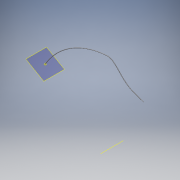
# Autodesk Inventor part: bumper_wire
Saved by Autodesk Inventor 2016 (Build 200138000, 138)
## iProperties
Created: 2016-02-23
Part Number: bumper_wire
Material: Generic
Document SubType Name: Modeling
Designer: jforce
Density: 1 g/cm^3
Appearance: Default
Author: jforce
Autodesk Inventor part; units mm, degrees
ref_plane "YZ Plane" through (0, 0, 0) normal (1, 0, 0) x (0, 1, 0)
ref_plane "XZ Plane" through (0, 0, 0) normal (0, 1, 0) x (-1, 0, 0)
ref_plane "XY Plane" through (0, 0, 0) normal (0, 0, 1) x (1, 0, 0)
sketch "Sketch1" plane through (0, 0, 0) normal (0, 0, 1) x (1, 0, 0)
  arc A0 (-6.4467, 81.7462) -> (71.0141, 41) centre (0, 0) ccw construction
  arc A1 (-6.4467, 81.7462) -> (-71.0141, 41) centre (0, 0) ccw
  line L0 (0, 0) -> (87.6874, 50.6264) construction
  line L1 (-50.8467, 0) -> (49.6534, 0) construction
  line L2 (0, 0) -> (-79.9103, 46.1363) construction
  line L3 (0, 0) -> (-7.0236, 89.0614) construction
  line L4 (-6.4467, 81.7462) -> (-3.5118, 81.9776) construction
  line L5 (-3.5118, 81.9776) -> (1.9145, 81.9776) construction
  line L6 (1.9145, 81.9776) -> (12.9687, 65.2245) construction
  line L7 (12.9687, 65.2245) -> (22.4637, 62.3445) construction
  line L8 (22.4637, 62.3445) -> (29.5777, 59.9957) construction
  line L9 (29.5777, 59.9957) -> (33.8283, 58.5923) construction
  spline S0 degree 4 poles (-6.4467, 81.7462) (-3.5118, 81.9776) (1.9145, 81.9776) (12.9687, 65.2245) (22.4637, 62.3445) (29.5777, 59.9957) (33.8283, 58.5923) knots 1 1 1 1 1 2 3 4 4 4 4 4
  dimension "d0" = 164
  dimension "d1" = 30
  dimension "d2" = 30
  constraints: 8 end point, 4 point on circle, 3 coincident, 3 point on line, 2 centre point, 2 horizontal, 1 perpendicular, 3 other
  measures "d0" diameter of A0
  measures "d1" angle of L0 L1
  measures "d2" angle of L2 L1
ref_plane "Work Plane1" through (-71.0141, 41, 0) normal (-0.5, -0.866, 0) x (0.866, -0.5, 0)
sketch "Sketch2" plane through (-71.0141, 41, 0) normal (-0.5, -0.866, 0) x (0.866, -0.5, 0)
  circle A0 centre (0, 0) radius 0.325
  point P0 (82, 0)
  dimension "d3" = 0.65
  constraints: 1 centre point
  measures "d3" diameter of A0
sweep "Sweep1" add profiles "Sketch2" path "Sketch1"
body "Solid1"
